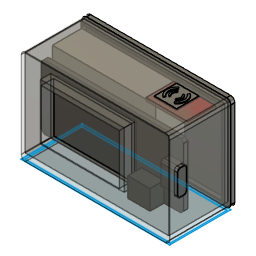
weather station (Autodesk Fusion 360 design; units mm, degrees)
Autodesk Fusion 360 part; units mm, degrees
sketch "Sketch1" plane through (0, 0, 0) normal (0, 1, 0) x (1, 0, 0)
  line L0 (0, 0) -> (51, 0)
  line L1 (51, 0) -> (51, -23)
  line L2 (51, -23) -> (0, -23)
  line L3 (0, -23) -> (0, 0)
  dimension "d1" = 51
  dimension "d2" = 23
  constraint horizontal L0
  constraint vertical L1
  constraint horizontal L2
  constraint vertical L3
  constraint coincident L0.start L3.end
  measures "d1" distance of L0.start L0.end
  measures "d2" distance of L0.start L2.end
extrude "Extrude1" add sketch "Sketch1" along normal blind 1.5 makes body 1
sketch "Sketch2" plane through (0, 1.5, 0) normal (0, 1, 0) x (-1, 0, 0)
  line L0 (0, 23) -> (-51, 23)
  line L1 (-51, 23) -> (-51, 0)
  line L2 (-51, 0) -> (0, 0)
  line L3 (0, 0) -> (0, 23)
  line L4 (0, 0) -> (-6, 0)
  line L5 (-6, 0) -> (-6, 2)
  line L6 (-6, 2) -> (0, 2)
  line L7 (0, 2) -> (0, 0)
  line L8 (-6, 2) -> (-34, 2)
  line L9 (-34, 2) -> (-34, 20)
  line L10 (-34, 20) -> (-6, 20)
  line L11 (-6, 20) -> (-6, 2)
  line L12 (-51, 23) -> (-44, 23)
  line L13 (-44, 23) -> (-36, 23)
  line L14 (-36, 23) -> (-36, 16)
  line L15 (-36, 16) -> (-44, 16)
  line L16 (-44, 16) -> (-44, 23)
  line L17 (-6, 2.5) -> (-34, 2.5)
  line L18 (-34, 2.5) -> (-34, 20.5)
  line L19 (-34, 20.5) -> (-6, 20.5)
  line L20 (-6, 20.5) -> (-6, 2.5)
  line L21 (-51, 11.5) -> (-39, 11.5)
  line L22 (-51, 11.5) -> (-51, 7)
  line L23 (-46, 7) -> (-52, 7)
  line L24 (-52, 7) -> (-52, 16)
  line L25 (-52, 16) -> (-46, 16)
  line L26 (-46, 16) -> (-46, 7)
  dimension "d5" = 6
  dimension "d6" = 2
  dimension "d7" = 28
  dimension "d8" = 18
  dimension "d9" = 7
  dimension "d10" = 8
  dimension "d11" = 7
  dimension "d16" = 4.5
  dimension "d17" = 6
  dimension "d18" = 9
  constraint horizontal L4
  constraint vertical L5
  constraint horizontal L6
  constraint vertical L7
  constraint coincident L2.end L3.start
  constraint horizontal L8
  constraint vertical L9
  constraint horizontal L10
  constraint vertical L11
  constraint coincident L0.end L1.start
  constraint perpendicular L1 L12
  constraint horizontal L13
  constraint vertical L14
  constraint horizontal L15
  constraint vertical L16
  constraint horizontal L17
  constraint vertical L18
  constraint horizontal L19
  constraint vertical L20
  constraint coincident L11 L17.start
  constraint midpoint L1 L21.start
  constraint perpendicular L1 L21
  constraint perpendicular L21 L22
  constraint horizontal L23
  constraint vertical L24
  constraint horizontal L25
  constraint vertical L26
  measures "d5" distance of L2.end L4.end
  measures "d6" distance of L2.end L6.end
  measures "d7" distance of L5.end L8.end
  measures "d8" distance of L5.end L10.end
  measures "d9" distance of L0.end L12.end
  measures "d10" distance of L12.end L13.end
  measures "d11" distance of L12.end L15.end
  measures "d16" distance of L21.start L22.end
  measures "d17" distance of L23.start L23.end
  measures "d18" distance of L23.start L25.end
extrude "Extrude2" add sketch "Sketch2" along normal blind 2.2 contours L9 L10 L11 L17 L18 L20 | L10 L18 L19 L20 bodies 1
extrude "Extrude3" add sketch "Sketch2" along normal blind 5 contours L0 L13 L14 L15 L16 bodies 1
extrude "Extrude4" add sketch "Sketch2" along normal blind 3.1 contours L1 L21 L25 L26 | L1 L22 L23 L24 L25 | L1 L21 L22 L23 L26 bodies 1
fillet "Fillet1" radius 1 2 edges at (49, 4.6, 16) (49, 4.6, 7) on bodies 1
fillet "Fillet2" radius 1 2 edges at (51.5, 1.5, 7) (51.5, 1.5, 16) on bodies 1
extrude "Extrude5" cut 1 faces at (15.3333, 3.7, 8.3333) along direction (0, -1, 0) blind 0.3 on bodies 1 bodies 1
extrude "Extrude6" cut 1 faces at (15.3333, 3.4, 8.3333) along direction (0, -1, 0) blind 0.5 on bodies 1 bodies 1
chamfer "Chamfer1" distance 1 angle 45 4 edges at (0, 0.75, 23) (0, 0.75, 0) (51, 0.75, 0) (51, 0.75, 23) on bodies 1
sketch "Sketch3" plane through (0, 0, 0) normal (0, 1, 0) x (1, 0, 0)
  line L0 (-2, 0) -> (-42, 0)
  line L1 (-42, 0) -> (-42, 29)
  line L2 (-42, 29) -> (-2, 29)
  line L3 (-2, 29) -> (-2, 0)
  dimension "d30" = 40
  dimension "d31" = 29
  constraint horizontal L0
  constraint vertical L1
  constraint horizontal L2
  constraint vertical L3
  measures "d30" distance of L0.start L0.end
  measures "d31" distance of L0.start L2.end
extrude "Extrude7" add sketch "Sketch3" along normal blind 10.5 separate body makes body 2
sketch "Sketch4" plane through (0, 0, 0) normal (0, 1, 0) x (1, 0, 0)
  line L0 (-5, -20) -> (-20, -20)
  line L1 (-20, -20) -> (-20, -10)
  line L2 (-20, -10) -> (-5, -10)
  line L3 (-5, -10) -> (-5, -20)
  dimension "d34" = 15
  dimension "d35" = 10
  constraint horizontal L0
  constraint vertical L1
  constraint horizontal L2
  constraint vertical L3
  measures "d34" distance of L0.start L0.end
  measures "d35" distance of L0.start L2.end
extrude "Extrude8" add sketch "Sketch4" along normal blind 1 separate body makes body 3
move_body "Move1" bodies 1 to x (1, 0, 0) y (0, 0, 1) z (0, -1, 0) at (0, 29, 0)
move_body "Move2" bodies 2 to x (1, 0, 0) y (0, 0, 1) z (0, -1, 0) at (0, 3, -12)
move_body "Move3" bodies 2 to x (1, 0, 0) y (0, 1, 0) z (0, 0, 1) at (43, 0, 0)
move_body "Move4" bodies 3 to x (1, 0, 0) y (0, 1, 0) z (0, 0, 1) at (55, 32, 0)
extrude "Extrude9" cut 1 faces at (41, 22.3333, -8.5) along direction (-1, 0, 0) blind 3 on bodies 2 bodies 2
move_body "Move5" bodies 3 to x (1, 0, 0) y (0, 1, 0) z (0, 0, 1) at (0, 0, -21)
sketch "Sketch5" plane through (0, 0, 0) normal (0, 1, 0) x (1, 0, 0)
  line L0 (-0.5, 13.5) -> (51.5, 13.5)
  line L1 (51.5, 13.5) -> (51.5, -6.8)
  line L2 (51.5, -6.8) -> (-0.5, -6.8)
  line L3 (-0.5, -6.8) -> (-0.5, 13.5)
  line L4 (52, -7.5) -> (-1.2407, -7.5)
  line L5 (-1.2407, -7.5) -> (-1.2407, 14.3963)
  line L6 (-1.2407, 14.3963) -> (52, 14.3963)
  line L7 (52, 14.3963) -> (52, -7.5)
  constraint horizontal L0
  constraint vertical L1
  constraint horizontal L2
  constraint vertical L3
  constraint horizontal L4
  constraint vertical L5
  constraint horizontal L6
  constraint vertical L7
extrude "Extrude10" add sketch "Sketch5" along normal blind 2 separate body contours L0 L1 L2 L3 | L4 L5 L6 L7 makes body 4
extrude "Extrude11" add sketch "Sketch5" along normal blind 34 bodies 4
sketch "Sketch6" plane through (0, 0, 7.5) normal (0, 0, 1) x (1, 0, 0)
  line L0 (-1.2407, 0) -> (52, 0)
  line L1 (52, 0) -> (52, 34)
  line L2 (52, 34) -> (-1.2407, 34)
  line L3 (-1.2407, 34) -> (-1.2407, 0)
  line L4 (6, 26.5) -> (34, 26.5)
  line L5 (34, 26.5) -> (34, 8.5)
  line L6 (34, 8.5) -> (6, 8.5)
  line L7 (6, 8.5) -> (6, 26.5)
  constraint horizontal L4
  constraint vertical L5
  constraint horizontal L6
  constraint vertical L7
extrude "Extrude12" cut sketch "Sketch6" against normal blind 2 contours L4 L5 L6 L7 bodies 4
extrude "Extrude13" add 1 faces at (16.8333, 12.6667, -13.5) along direction (0, 0, 1) blind 1 on bodies 4 bodies 4
extrude "Extrude14" add 1 faces at (51.5, 12.6667, -6.0667) along direction (-1, 0, 0) blind 0.5 on bodies 4 bodies 4
sketch "Sketch7" plane through (52, 0, 0) normal (1, 0, 0) x (0, 0, -1)
  line L0 (-7.5, 0) -> (14.3963, 0)
  line L1 (14.3963, 0) -> (14.3963, 34)
  line L2 (14.3963, 34) -> (-7.5, 34)
  line L3 (-7.5, 34) -> (-7.5, 0)
  line L4 (-4.6, 22) -> (-1.5, 22)
  line L5 (-1.5, 22) -> (-1.5, 13)
  line L6 (-1.5, 13) -> (-4.6, 13)
  line L7 (-4.6, 13) -> (-4.6, 22)
  constraint horizontal L4
  constraint vertical L5
  constraint horizontal L6
  constraint vertical L7
extrude "Extrude15" cut sketch "Sketch7" against normal blind 2 contours L4 L5 L6 L7 bodies 4
move_face "OffsetFaces1" offset -0.2 4 faces at (51.6667, 19, 1.5) (51.6667, 16, 4.6) (51.6667, 13, 2.5333) (51.6667, 22, 3.5667) on bodies 4
fillet "Fillet3" radius 1 4 edges at (51.5, 22.2, 4.8) (51.5, 22.2, 1.3) (51.5, 12.8, 1.3) (51.5, 12.8, 4.8) on bodies 4
sketch "Sketch8" plane through (0, 34, 0) normal (0, 1, 0) x (-1, 0, 0)
  line L0 (-51, 6.8) -> (0.5, 6.8)
  line L1 (0.5, 6.8) -> (0.5, -12.5)
  line L2 (0.5, -12.5) -> (-51, -12.5)
  line L3 (-51, -12.5) -> (-51, 6.8)
  line L4 (-52, -14.3963) -> (1.2407, -14.3963)
  line L5 (1.2407, -14.3963) -> (1.2407, 7.5)
  line L6 (1.2407, 7.5) -> (-52, 7.5)
  line L7 (-52, 7.5) -> (-52, -14.3963)
  line L8 (1.2407, -14.3963) -> (-52, -14.3963)
  line L9 (-52, -14.3963) -> (-52, 7.5)
  line L10 (-52, 7.5) -> (1.2407, 7.5)
  line L11 (1.2407, 7.5) -> (1.2407, -14.3963)
  constraint horizontal L8
  constraint vertical L9
  constraint horizontal L10
  constraint vertical L11
  constraint coincident L6.end L7.start
  constraint coincident L4.end L5.start
extrude "Extrude16" add sketch "Sketch8" against normal blind 1 contours L0 L1 L2 L3 | L4 L5 L6 L7 L8 L9 L10 L11 bodies 4
sketch "Sketch9" plane through (0, 34, 0) normal (0, 1, 0) x (-1, 0, 0)
  line L0 (-52, -14.3963) -> (1.2407, -14.3963)
  line L1 (1.2407, -14.3963) -> (1.2407, 7.5)
  line L2 (1.2407, 7.5) -> (-52, 7.5)
  line L3 (-52, 7.5) -> (-52, -14.3963)
  line L4 (-37, -10) -> (-45, -10)
  line L5 (-45, -10) -> (-45, -2)
  line L6 (-45, -2) -> (-37, -2)
  line L7 (-37, -2) -> (-37, -10)
  circle A0 centre (-41, -6) radius 3.5
  circle A1 centre (-41, -6) radius 2.75
  circle A2 centre (-41, -6) radius 2
  circle A3 centre (-41, -6) radius 1.5
  line L8 (-38.5, -9.5) -> (-41, -6)
  line L9 (-41, -6) -> (-38.5, -2.5)
  line L10 (-38.5, -9.5) -> (-43.5, -9.5)
  line L11 (-43.5, -9.5) -> (-41, -6)
  line L12 (-41, -6) -> (-43.5, -2.5)
  line L13 (-43.5, -2.5) -> (-38.5, -2.5)
  dimension "d57" = 7
  dimension "d58" = 5.5
  dimension "d59" = 4
  dimension "d60" = 3
  constraint horizontal L4
  constraint vertical L5
  constraint horizontal L6
  constraint vertical L7
  constraint concentric A0 A1
  constraint concentric A0 A2
  constraint concentric A2 A3
  constraint coincident A0.centre A1.centre
  constraint parallel L4 L10
  constraint parallel L9 L11
  constraint parallel L10 L13
  measures "d57" diameter of A0
  measures "d58" diameter of A1
  measures "d59" diameter of A2
  measures "d60" diameter of A3
extrude "Extrude17" cut sketch "Sketch9" against normal blind 0.4 contours L4 L5 L6 L7 | A0 A1 L8 L9 | A0 A1 L9 L12 | A0 L9 L13 | A0 L8 L10 | A0 A1 L8 L11 | A0 L12 L13 | A1 A2 L9 L12 | A1 A2 L8 L9 | A0 L10 L11 | A1 A2 L8 L11 | A0 A1 L11 L12 | A1 A2 L11 L12 | A2 A3 L9 L12 | A2 A3 L8 L9 | A2 A3 L8 L11 | A2 A3 L11 L12 | A3 L9 L12 | A3 L8 L9 | A3 L8 L11 | A3 L11 L12 bodies 4
extrude "Extrude18" add sketch "Sketch9" against normal blind 0.3 separate body contours L4 L5 L6 L7 | A0 A1 L8 L9 | A0 A1 L9 L12 | A0 L9 L13 | A0 L8 L10 | A0 A1 L8 L11 | A0 L12 L13 | A1 A2 L9 L12 | A1 A2 L8 L9 | A0 L10 L11 | A1 A2 L8 L11 | A0 A1 L11 L12 | A1 A2 L11 L12 | A2 A3 L9 L12 | A2 A3 L8 L9 | A2 A3 L8 L11 | A2 A3 L11 L12 | A3 L9 L12 | A3 L8 L9 | A3 L8 L11 | A3 L11 L12 makes body 5
extrude "Extrude19" add sketch "Sketch9" along normal blind 0.3 contours A0 A1 L8 L9 | A0 A1 L11 L12 | A2 A3 L8 L9 | A2 A3 L11 L12 bodies 5
extrude "Extrude20" cut 1 faces at (34.2531, 22.6667, -14.3963) along direction (0, 0, 1) blind 2 on bodies 4 bodies 4
extrude "Extrude21" add 1 faces at (33.9198, 0.6667, -12.3963) along direction (0, 0, -1) blind 2 on bodies 4 bodies 4
fillet "Fillet4" radius 1.5 4 edges at (52, 34, -3.4481) (-1.2407, 34, -3.4481) (-1.2407, 0, -3.4481) (52, 0, -3.4481) on bodies 4
sketch "Sketch10" plane through (0, 0, -14.3963) normal (0, 0, -1) x (-1, 0, 0)
  line L0 (-51, 33) -> (0.5, 33)
  line L1 (0.5, 33) -> (0.5, 2)
  line L2 (0.5, 2) -> (-51, 2)
  line L3 (-51, 2) -> (-51, 33)
  arc A0 (-52, 1.5) -> (-50.5, 0) centre (-50.5, 1.5) ccw
  line L4 (-50.5, 0) -> (-0.2593, 0)
  arc A1 (-0.2593, 0) -> (1.2407, 1.5) centre (-0.2593, 1.5) ccw
  line L5 (1.2407, 1.5) -> (1.2407, 32.5)
  arc A2 (1.2407, 32.5) -> (-0.2593, 34) centre (-0.2593, 32.5) ccw
  line L6 (-0.2593, 34) -> (-50.5, 34)
  arc A3 (-50.5, 34) -> (-52, 32.5) centre (-50.5, 32.5) ccw
  line L7 (-52, 32.5) -> (-52, 1.5)
  line L8 (-50.5, 34) -> (-0.2574, 34)
  line L9 (1.2426, 32.5) -> (1.2426, 1.4966)
  line L10 (-0.2574, -0.0034) -> (-50.5, -0.0034)
  line L11 (-52, 1.4966) -> (-52, 32.5)
  arc A4 (-52, 1.4966) -> (-50.5, -0.0034) centre (-50.5, 1.4966) ccw
  arc A5 (-0.2574, -0.0034) -> (1.2426, 1.4966) centre (-0.2574, 1.4966) ccw
  arc A6 (1.2426, 32.5) -> (-0.2574, 34) centre (-0.2574, 32.5) ccw
  arc A7 (-50.5, 34) -> (-52, 32.5) centre (-50.5, 32.5) ccw
  line L12 (-51, 33) -> (0.5, 33)
  line L13 (0.5, 33) -> (0.5, 2)
  line L14 (0.5, 2) -> (-51, 2)
  line L15 (-51, 2) -> (-51, 33)
  line L16 (-0.233, 2.722) -> (-50.2347, 2.722)
  line L17 (-50.2347, 2.722) -> (-50.2347, 32.2528)
  line L18 (-50.2347, 32.2528) -> (-0.233, 32.2528)
  line L19 (-0.233, 32.2528) -> (-0.233, 2.722)
  dimension "d73" = 1.5
  constraint horizontal L8
  constraint vertical L9
  constraint horizontal L10
  constraint vertical L11
  constraint tangent L10 A4
  constraint tangent L11 A4
  constraint tangent L9 A5
  constraint tangent L10 A5
  constraint equal A4 A5
  constraint tangent L8 A6
  constraint tangent L9 A6
  constraint equal A4 A6
  constraint tangent L8 A7
  constraint tangent L11 A7
  constraint equal A4 A7
  constraint horizontal L12
  constraint vertical L13
  constraint horizontal L14
  constraint vertical L15
  constraint coincident L1.end L2.start
  constraint coincident L0.start L3.end
  constraint horizontal L16
  constraint vertical L17
  constraint horizontal L18
  constraint vertical L19
  measures "d73" radius of A4
extrude "Extrude22" add sketch "Sketch10" along normal blind 2 separate body contours L0 L1 L2 L3 L12 L13 L14 L15 | A0 L4 A1 L5 A2 L6 A3 L7 L8 L9 L11 A6 A7 | A0 L4 A1 L10 A4 A5 | L16 L17 L18 L19 makes body 6
extrude "Extrude23" add sketch "Sketch10" against normal blind 2 contours L0 L1 L2 L3 L12 L13 L14 L15 bodies 6
extrude "Extrude24" cut 1 faces at (50.7449, 22.4176, -12.3963) along direction (0, 0, -1) blind 0.5 on bodies 6 bodies 6
chamfer "Chamfer2" distance 0.35 angle 45 4 edges at (25.25, 33, -12.8963) (51, 17.5, -12.8963) (25.25, 2, -12.8963) (-0.5, 17.5, -12.8963) on bodies 6
extrude "Extrude25" cut 1 faces at (33.7531, 11.3333, -16.3963) along direction (0, 0, 1) blind 1 on bodies 6 bodies 6
extrude "Extrude26" add 1 faces at (33.7531, 11.3333, -15.3963) along direction (0, 0, -1) blind 0.5 on bodies 6 bodies 6
sketch "Sketch11" plane through (0, 0, 6.8) normal (0, 0, -1) x (-1, 0, 0)
  line L0 (-34, 8.5) -> (-34, 26.5)
  line L1 (-34, 26.5) -> (-6, 26.5)
  line L2 (-6, 26.5) -> (-6, 8.5)
  line L3 (-6, 8.5) -> (-34, 8.5)
  line L4 (0.5, 33) -> (-51, 33)
  line L5 (-51, 33) -> (-51, 2)
  line L6 (-51, 2) -> (0.5, 2)
  line L7 (0.5, 2) -> (0.5, 33)
  line L8 (-35, 27.5) -> (-5, 27.5)
  line L9 (-5, 27.5) -> (-5, 7.5)
  line L10 (-5, 7.5) -> (-35, 7.5)
  line L11 (-35, 7.5) -> (-35, 27.5)
  constraint horizontal L8
  constraint vertical L9
  constraint horizontal L10
  constraint vertical L11
extrude "Extrude27" add sketch "Sketch11" along normal blind 4 contours L8 L9 L10 L11 bodies 4
extrude "Extrude28" cut 1 faces at (24.6667, 27.1667, 2.8) along direction (0, 0, 1) blind 0.3 on bodies 4 bodies 4
named bodies: "ESP32", "Battery", "Touch", "Case", "Touch indicator", "Lid"
